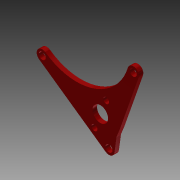
# Autodesk Inventor part: OutlineSketch1
Saved by Autodesk Inventor 2013 (Build 170138000, 138)
## iProperties
Created: 2013-06-03
Part Number: OutlineSketch1
Material: Aluminum 6061
Document SubType Name: Modeling
Designer: mvarma
Density: 2.71 g/cm^3
Author: mvarma
Autodesk Inventor part; units mm, degrees
ref_plane "YZ Plane" through (0, 0, 0) normal (1, 0, 0) x (0, 1, 0)
ref_plane "XZ Plane" through (0, 0, 0) normal (0, 1, 0) x (-1, 0, 0)
ref_plane "XY Plane" through (0, 0, 0) normal (0, 0, 1) x (1, 0, 0)
sketch "Sketch1" plane through (0, 0, 0) normal (0, 0, 1) x (1, 0, 0)
  line L0 (0, 0) -> (304.8, 0) construction
  line L1 (304.8, 0) -> (304.8, 50.8) construction
  line L2 (304.8, 50.8) -> (0, 50.8) construction
  line L3 (0, 50.8) -> (0, 0) construction
  circle A0 centre (152.4, 23.8125) radius 6.35 construction
  circle A1 centre (152.4, 23.8125) radius 34.29 construction
  circle A2 centre (152.4, 23.8125) radius 22.225 construction
  line L4 (152.4, 23.8125) -> (139.52, 61.741) construction
  circle A3 centre (139.52, 61.741) radius 9.525 construction
  circle A4 centre (139.52, 61.741) radius 17.78 construction
  circle A5 centre (91.5619, 85.09) radius 31.75 construction
  circle A6 centre (163.3424, 109.4657) radius 31.75 construction
  line L5 (0, 50.8) -> (0, 53.34) construction
  line L6 (0, 53.34) -> (304.8, 53.34) construction
  line L7 (304.8, 53.34) -> (304.8, 50.8) construction
  circle A7 centre (139.52, 61.741) radius 21.59 construction
  circle A8 centre (152.4, 23.8125) radius 46.99 construction
  circle A9 centre (152.4, 23.8125) radius 50.8 construction
  arc A10 (86.3865, 79.4564) -> (92.4363, 92.6899) centre (91.5619, 85.09) ccw construction
  circle A11 centre (163.3424, 109.4657) radius 7.65 construction
  circle A12 centre (163.3424, 109.4657) radius 9.1 construction
  circle A13 centre (139.52, 61.741) radius 22.9 construction
  line L8 (86.3865, 79.4564) -> (124.0276, 44.8769) construction
  line L9 (170.8782, 108.1486) -> (162.078, 57.7984) construction
  line L10 (92.4363, 92.6899) -> (91.5619, 85.09) construction
  line L11 (91.5619, 85.09) -> (86.3865, 79.4564) construction
  arc A14 (128.9499, 92.8673) -> (131.407, 97.9722) centre (127.6738, 96.6252) ccw
  circle A15 centre (127.6738, 96.6252) radius 7.9375 construction
  line L12 (92.4363, 92.6899) -> (126.7664, 88.7398) construction
  line L13 (133.1953, 90.9229) -> (158.0208, 114.9615) construction
  line L14 (158.0208, 114.9615) -> (163.3424, 109.4657) construction
  line L15 (170.8782, 108.1486) -> (163.3424, 109.4657) construction
  line L16 (139.52, 61.741) -> (127.6738, 96.6252) construction
  line L17 (91.5619, 85.09) -> (163.3424, 109.4657) construction
  line L18 (152.4, 23.8125) -> (91.5619, 85.09) construction
  line L19 (152.4, 23.8125) -> (163.3424, 109.4657) construction
  circle A16 centre (127.6738, 96.6252) radius 9.2075 construction
  circle A17 centre (127.6738, 96.6252) radius 6.1595 construction
  arc A18 (92.4363, 92.6899) -> (86.3865, 79.4564) centre (91.5619, 85.09) ccw construction
  circle A19 centre (163.3424, 109.4657) radius 25.4 construction
  line L20 (104.7627, 113.9656) -> (78.361, 56.2144) construction
  circle A20 centre (91.5619, 85.09) radius 25.4 construction
  line L21 (104.4015, 107.0791) -> (92.7013, 84.5343) construction
  line L22 (81.0012, 61.9895) -> (90.3961, 85.5882) construction
  arc A21 (100.6718, 111.3992) -> (98.9102, 106.9744) centre (99.791, 109.1868) ccw construction
  arc A22 (103.3046, 104.9655) -> (105.4983, 109.1926) centre (104.4015, 107.0791) ccw construction
  arc A23 (103.3046, 104.9655) -> (98.9102, 106.9744) centre (81.0012, 61.9895) ccw construction
  line L23 (99.791, 109.1868) -> (100.6718, 111.3992) construction
  line L24 (104.4015, 107.0791) -> (105.4983, 109.1926) construction
  arc A24 (105.4983, 109.1926) -> (100.6718, 111.3992) centre (81.0012, 61.9895) ccw construction
  arc A25 (88.0213, 75.5164) -> (97.3814, 93.5522) centre (92.7013, 84.5343) ccw construction
  line L25 (90.3961, 85.5882) -> (99.791, 109.1868) construction
  line L26 (92.7013, 84.5343) -> (81.0012, 61.9895) construction
  arc A26 (88.0213, 75.5164) -> (86.6381, 76.1487) centre (81.0012, 61.9895) ccw construction
  arc A27 (97.3814, 93.5522) -> (94.1541, 95.0276) centre (81.0012, 61.9895) ccw construction
  arc A28 (94.1541, 95.0276) -> (86.6381, 76.1487) centre (90.3961, 85.5882) ccw construction
  line L27 (163.3424, 109.4657) -> (140.8985, 121.3583) construction
  line L28 (163.3424, 109.4657) -> (185.7862, 97.5731) construction
  circle A29 centre (139.52, 61.741) radius 26.71 construction
  circle A30 centre (152.4, 23.8125) radius 11.176 construction
  line L29 (152.4, 23.8125) -> (158.5256, 5.7742) construction
  circle A31 centre (152.4, 23.8125) radius 5.5065
  line L30 (156.5338, 34.1959) -> (148.2662, 13.4291) construction
  circle A32 centre (156.5338, 34.1959) radius 2.1082
  circle A33 centre (148.2662, 13.4291) radius 2.1082
  arc A34 (166.3874, 21.8643) -> (163.8992, 15.6142) centre (152.4, 23.8125) ccw
  circle A35 centre (111.304, 39.007) radius 9.525 construction
  circle A36 centre (175.745, 60.8903) radius 9.525 construction
  arc A37 (113.6108, 42.2365) -> (109.0199, 35.7614) centre (111.304, 39.007) ccw
  arc A38 (179.4939, 59.5878) -> (171.9486, 62.0473) centre (175.745, 60.8903) ccw
  arc A39 (157.2494, 9.5322) -> (156.2414, 2.5286) centre (158.5256, 5.7742) ccw
  line L31 (152.4, 23.8125) -> (165.1433, 18.7393) construction
  line L32 (166.3874, 21.8643) -> (163.8992, 15.6142)
  arc A40 (163.8992, 15.6142) -> (166.3874, 21.8643) centre (152.4, 23.8125) ccw construction
  line L33 (163.8992, 15.6142) -> (162.4566, 5.2282)
  line L34 (156.2414, 2.5286) -> (109.0199, 35.7614)
  line L35 (166.3874, 21.8643) -> (179.4939, 59.5878)
  arc A41 (123.8923, 95.4203) -> (128.9499, 92.8673) centre (127.6738, 96.6252) ccw
  arc A42 (131.407, 97.9722) -> (123.8923, 95.4203) centre (127.6738, 96.6252) ccw
  arc A43 (131.202, 98.5513) -> (131.407, 97.9722) centre (178.6686, 115.0239) ccw
  arc A44 (162.4566, 5.2282) -> (157.2494, 9.5322) centre (158.5256, 5.7742) ccw
  arc A45 (156.2414, 2.5286) -> (162.4566, 5.2282) centre (158.5256, 5.7742) ccw
  circle A46 centre (135.6607, 73.1057) radius 37.9355
  point P0 (102.1225, 108.1905)
  point P1 (145.0256, 46.8513)
  dimension "d1" = 50.8
  dimension "d3" = 23.8125
  dimension "d4" = 152.4
  dimension "d7" = 68.58
  dimension "d8" = 44.45
  dimension "d9" = 19.05
  dimension "d10" = 35.56
  dimension "d11" = 40.0558
  dimension "d12" = 63.5
  dimension "d13" = 63.5
  dimension "d15" = 2.54
  dimension "d16" = 304.8
  dimension "d17" = 43.18
  dimension "d18" = 93.98
  dimension "d19" = 101.6
  dimension "d21" = 15.3
  dimension "d22" = 15.3
  dimension "d24" = 18.2
  dimension "d29" = 45.8
  dimension "d30" = 143.991
  dimension "d31" = 7.9375
  dimension "d32" = 15.875
  dimension "d33" = 143.991
  dimension "d35" = 18.415
  dimension "d37" = 12.319
  dimension "d40" = 50.8
  dimension "d42" = 18.004
  dimension "d43" = 18.004
  dimension "d44" = 50.8
  dimension "d75" = 2.86
  dimension "d80" = 4.7625
  dimension "d82" = 4.7625
  dimension "d83" = 50.8
  dimension "d84" = 50.8
  dimension "d97" = 48.4188
  dimension "d99" = 20.32
  dimension "d101" = 25.4
  dimension "d102" = 25.4
  dimension "d103" = 10.16
  dimension "d105" = 18.004
  dimension "d106" = 18.004
  dimension "d107" = 53.42
  dimension "d149" = 22.352
  dimension "d152" = 180
  dimension "d163" = 11.013
  dimension "d190" = 12.7
  dimension "d191" = 4.2164
  dimension "d192" = 4.2164
  dimension "d209" = 28.2448
  dimension "d210" = 19.05
  dimension "d211" = 19.05
  dimension "d212" = 7.9375
  dimension "d214" = 19.05
  dimension "d215" = 7.9375
  dimension "d216" = 13.716
  dimension "d232" = 3.9688
  constraints: 74 end point, 59 point on circle, 47 centre point, 31 coincident, 24 tangent, 10 point on line, 7 collinear, 7 perpendicular, 4 parallel, 3 midpoint, 1 horizontal, 1 symmetric about line, 2 other
  measures "d1" distance of L1.end L0.end
  measures "d3" distance from line of L0 A0.centre
  measures "d4" distance from line of L3 A0.centre
  measures "d7" diameter of A1
  measures "d8" diameter of A2
  measures "d9" diameter of A3
  measures "d10" diameter of A4
  measures "d11" distance of L4.start L4.end
  measures "d12" diameter of A5
  measures "d13" diameter of A6
  measures "d15" distance of L2.end L5.end
  measures "d16" distance of L0.end L0.start
  measures "d17" diameter of A7
  measures "d18" diameter of A8
  measures "d19" diameter of A9
  measures "d21" diameter of A10
  measures "d22" diameter of A11
  measures "d24" diameter of A12
  measures "d29" diameter of A13
  measures "d30" angle of L11 L10
  measures "d31" diameter of A14
  measures "d32" diameter of A15
  measures "d33" angle of L15 L14
  measures "d35" diameter of A16
  measures "d37" diameter of A17
  measures "d40" diameter of A19
  measures "d42" angle of L10 L20
  measures "d43" angle of L11 L20
  measures "d44" diameter of A20
  measures "d75" angle of L20 L21
  measures "d80" diameter of A21
  measures "d82" diameter of A22
  measures "d83" distance of L22.start L25.end
  measures "d84" distance of L21.start L22.start
  measures "d97" radius of A23
  measures "d99" diameter of A25
  measures "d101" distance of L22.start L22.end
  measures "d102" distance of L21.end L22.start
  measures "d103" radius of A28
  measures "d105" angle of L27 L14
  measures "d106" angle of L28 L15
  measures "d107" diameter of A29
  measures "d149" diameter of A30
  measures "d152" angle of L29 L4
  measures "d163" diameter of A31
  measures "d190" diameter of A0
  measures "d191" diameter of A32
  measures "d192" diameter of A33
  measures "d209" diameter of A34
  measures "d210" diameter of A35
  measures "d211" diameter of A36
  measures "d212" diameter of A37
  measures "d214" distance of A0.centre L29.end
  measures "d215" diameter of A39
  measures "d216" distance of L31.start L31.end
  measures "d232" radius of A38
extrude "Extrusion3" add sketch "Sketch1" along normal blind 3.175 contours L32 A34 | A34 A46 A38 L35 | A34 L33 A44 A39 L34 A37 A46 | A45 A39 A44
hole "Hole3" at (81.0012, 61.9895, 0) at (185.7862, 97.5731, 0) at (127.6738, 96.6252, 0) at (111.304, 39.007, 0) at (175.745, 60.8903, 0) at (158.5256, 5.7742, 0) direction (0, 0, 1) diameter 4.9784 end through all clearance for "Socket Head Cap Screw" size "#10" standard "Ansi Unified Screw Threads"
fillet "Fillet3" radius 3.175 2 edges at (166.3874, 21.8643, 1.5875) (163.8992, 15.6142, 1.5875)
equation "\"d8\" = Gear35tPD"
equation "\"d9\" = Gear15tPD"
equation "\"d10\" = Gear28tPD"
equation "\"d11\" = 0.5 * Gear48tPD + 0.5 * Gear15tPD + MeshingClearance"
equation "\"d12\" = CimOD"
equation "\"d13\" = CimOD"
equation "\"d17\" = Gear28tPD + ClearanceDiameter"
equation "\"d18\" = WheelOD"
equation "\"d19\" = WheelClearance"
equation "\"Pulley48tPD\" = 45.8"
equation "\"Pulley19tPD\" = 18.2"
equation "\"Pulley16tPD\" = 15.3"
equation "\"Gear15tPD\" = 19.05"
equation "\"Gear35tPD\" = 44.45"
equation "\"Gear48tPD\" = 60.96"
equation "\"Gear28tPD\" = 35.56"
equation "\"BearingLargeOD\" = 28.575"
equation "\"BearingSmallOD\" = 22.225"
equation "\"MeshingClearance\" = 0.0508"
equation "\"CimOD\" = 63.5"
equation "\"WheelOD\" = 93.98"
equation "\"ClearanceDiameter\" = 7.62"
equation "\"WheelClearance\" = 101.6"
equation "\"TensioningBearingID\" = 6.35"
equation "\"TensioningBearingOD\" = 15.875"
equation "\"SpingClipClearance\" = 8.89"
equation "\"Pi\" = 79.79645"
equation "\"Pulley56tPD\" = 53.5"
equation "\"BearingXLargeOD\" = 34.925"
body "Solid3"
